oldleg (Autodesk Fusion 360 design; units mm, degrees)
Autodesk Fusion 360 part; units mm, degrees
note: some values were not read from the file. Chosen so that the rebuilt part matches the saved one: which bodies a step acts on; which pieces of a blend or face edit are solid.
sketch "Sketch1" plane through (0, 0, 0) normal (0, 0, 1) x (1, 0, 0)
  line L0 (60, 0) -> (45, 0)
  line L1 (45, 0) -> (45, 20)
  line L2 (45, 20) -> (60, 20)
  line L3 (60, 20) -> (60, 0)
  circle A0 centre (52.5, 7.5) radius 3.75
  line L4 (0, 120) -> (15, 120)
  line L5 (15, 120) -> (15, 100)
  line L6 (15, 100) -> (0, 100)
  line L7 (0, 100) -> (0, 120)
  circle A1 centre (7.5, 112.5) radius 3.75
  line L8 (0, 60) -> (60, 60)
  spline S0 degree 2 poles (0, 100) (0, 75) (20, 60) knots 0 0 0 4.583939 4.583939 4.583939 weights 1 0.818182 1
  line L9 (30, 30) -> (30, 90)
  spline S1 degree 2 poles (15, 100) (15, 80) (40, 60) knots 0 0 0 4.88998 4.88998 4.88998 weights 1 1.5 1
  spline S2 degree 2 poles (45, 20) (45, 40) (20, 60) knots 0 0 0 4.88998 4.88998 4.88998 weights 1 1.5 1
  spline S3 degree 2 poles (60, 20) (60, 45) (40, 60) knots 0 0 0 4.583939 4.583939 4.583939 weights 1 0.818182 1
  line L10 (60, 87.5) -> (0, 87.5)
  line L11 (0, 87.5) -> (0, 32.5)
  line L12 (0, 32.5) -> (60, 32.5)
  line L13 (60, 32.5) -> (60, 87.5)
  line L14 (60, 87.5) -> (0, 32.5) construction
  line L15 (0, 87.5) -> (60, 32.5) construction
  point P0 (30, 60)
  dimension "d3" = 15
  dimension "d4" = 20
  dimension "d5" = 7.5
  dimension "d8" = 15
  dimension "d9" = 20
  dimension "d10" = 7.5
  dimension "d20" = 120
  dimension "d21" = 60
  dimension "d25" = 80
  dimension "d26" = 0
  dimension "d27" = 45
  dimension "d28" = 7.5
  dimension "d29" = 7.5
  dimension "d30" = 7.5
  dimension "d31" = 7.5
  dimension "d32" = 30
  dimension "d33" = 60
  dimension "d54" = 60
  dimension "d55" = 55
  constraint horizontal L0
  constraint vertical L1
  constraint horizontal L2
  constraint vertical L3
  constraint horizontal L4
  constraint vertical L5
  constraint horizontal L6
  constraint vertical L7
  constraint horizontal L8
  constraint coincident L8 S0.end
  constraint vertical L9
  constraint coincident L8 S1.end
  constraint horizontal L10
  constraint perpendicular L10 L11
  constraint parallel L10 L12
  constraint parallel L11 L13
  constraint coincident L14 P0
  constraint coincident L15 P0
  constraint midpoint L8 P0
  measures "d3" distance of L0.start L0.end
  measures "d4" distance of L0.start L2.end
  measures "d5" diameter of A0
  measures "d8" distance of L4.start L4.end
  measures "d9" distance of L4.start L6.end
  measures "d10" diameter of A1
  measures "d20" distance of L0 L4
  measures "d21" distance of L3 L7
  measures "d25" distance of L2 L6
  measures "d26" distance of origin L0
  measures "d27" distance of origin L1
  measures "d28" distance of L1 A0.centre
  measures "d29" distance of L0 A0.centre
  measures "d30" distance of L4 A1.centre
  measures "d31" distance of L7 A1.centre
  measures "d32" distance of origin L9
  measures "d33" distance of origin L8
  measures "d54" distance of L11.end L12.end
  measures "d55" distance of L10.end L11.end
extrude "Extrude1" add sketch "Sketch1" along normal blind 35 contours L0 L1 L2 L3 makes body 1
extrude "Extrude2" add sketch "Sketch1" along normal blind 35 separate body contours L4 L5 L6 L7 makes body 2
fillet "Fillet1" radius 7.5 2 edges at (60, 0, 17.5) (45, 0, 17.5) on bodies 1
fillet "Fillet2" radius 7.5 2 edges at (15, 120, 17.5) (0, 120, 17.5) on bodies 2
sketch "Sketch2" plane through (0, 0, 0) normal (0, 1, 0) x (1, 0, 0)
  line L0 (45, 0) -> (60, 0)
  line L1 (60, 0) -> (60, -35)
  line L2 (60, -35) -> (45, -35)
  line L3 (45, -35) -> (45, 0)
  line L4 (60, -10) -> (45, -10)
  line L5 (45, -10) -> (45, -25)
  line L6 (45, -25) -> (60, -25)
  line L7 (60, -25) -> (60, -10)
  line L8 (60, -10) -> (45, -25) construction
  line L9 (45, -10) -> (60, -25) construction
  point P0 (52.5, -17.5)
  dimension "d42" = 15
  dimension "d43" = 15
  constraint horizontal L0
  constraint vertical L1
  constraint horizontal L2
  constraint vertical L3
  constraint horizontal L4
  constraint perpendicular L4 L5
  constraint parallel L4 L6
  constraint parallel L5 L7
  constraint coincident L1 L4.start
  constraint coincident L8 P0
  constraint coincident L9 P0
  measures "d42" distance of L0.start L0.end
  measures "d43" distance of L5.end L6.end
extrude "Extrude3" cut sketch "Sketch2" along normal blind 15 contours L1 L3 L4 L5 L6 L7 bodies 1
sketch "Sketch4" plane through (0, 100, 0) normal (0, -1, 0) x (1, 0, 0)
  line L0 (0, 0) -> (15, 0)
  line L1 (15, 0) -> (15, 35)
  line L2 (15, 35) -> (0, 35)
  line L3 (0, 35) -> (0, 0)
  line L4 (0, 0) -> (15, 0)
  line L5 (15, 0) -> (15, 35)
  line L6 (15, 35) -> (0, 35)
  line L7 (0, 35) -> (0, 0)
  line L8 (15, 10) -> (0, 10)
  line L9 (0, 10) -> (0, 25)
  line L10 (0, 25) -> (15, 25)
  line L11 (15, 25) -> (15, 10)
  line L12 (15, 10) -> (0, 25) construction
  line L13 (0, 10) -> (15, 25) construction
  point P0 (7.5, 17.5)
  dimension "d46" = 15
  dimension "d47" = 15
  constraint horizontal L4
  constraint vertical L5
  constraint horizontal L6
  constraint vertical L7
  constraint coincident L1.end L2.start
  constraint coincident L0.start L3.end
  constraint horizontal L8
  constraint perpendicular L8 L9
  constraint parallel L8 L10
  constraint parallel L9 L11
  constraint coincident L12 P0
  constraint coincident L13 P0
  measures "d46" distance of L9.end L10.end
  measures "d47" distance of L8.end L9.end
extrude "Extrude4" cut sketch "Sketch4" against normal blind 28 contours L1 L3 L5 L7 L8 L9 L10 L11 bodies 2 makes body 3 at (11.1756, 113.243, 3.3333)
extrude "Extrude5" add sketch "Sketch4" against normal blind 5 contours L1 L3 L5 L7 L8 L9 L10 L11 bodies 2 3
extrude "Extrude6" add sketch "Sketch1" along normal blind 35 contours L2 S2 S3 L12 | L8 L9 S2 S3 L12 | L8 L9 S1 | L8 L9 S2 | L8 S0 L9 S1 L10 | L6 S0 S1 L10 bodies 1 2
extrude "Extrude7" add sketch "Sketch1" along normal blind 40 contours L8 L9 S2 S3 L12 | L8 L9 S1 | L8 L9 S2 | L8 S0 L9 S1 L10 bodies 1
fillet "Fillet3" radius 18 4 edges at (50.8357, 32.5, 35) (50.8357, 32.5, 40) (9.1643, 87.5, 35) (9.1643, 87.5, 40) on bodies 1
extrude "Extrude8" cut sketch "Sketch1" along normal blind 25 contours L8 L9 S2 S3 L12 | L8 L9 S1 | L8 L9 S2 | L8 S0 L9 S1 L10 bodies 1
fillet "Fillet4" radius 15 4 edges at (50.8357, 32.5, 25) (9.1643, 87.5, 25) (9.1643, 87.5, 0) (50.8357, 32.5, 0) on bodies 1
